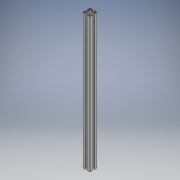
# Autodesk Inventor part: Alu_Proil_40
Saved by Autodesk Inventor 2019 (Build 230136000, 136)
## iProperties
Created: 2016-05-09
Part Number: Alu_Proil_40
Material: Generic
Document SubType Name: Modeling
Designer: Alfa
Density: 1 g/cm^3
Appearance: Default
Author: Alfa
Autodesk Inventor part; units mm, degrees
ref_plane "YZ Plane" through (0, 0, 0) normal (1, 0, 0) x (0, 1, 0)
ref_plane "XZ Plane" through (0, 0, 0) normal (0, 1, 0) x (-1, 0, 0)
ref_plane "XY Plane" through (0, 0, 0) normal (0, 0, 1) x (1, 0, 0)
sketch "Sketch1" plane through (0, 0, 0) normal (0, 0, 1) x (1, 0, 0)
  circle A0 centre (0, 0) radius 3.4
  line L0 (12.55, 11.55) -> (17.5, 11.55)
  arc A1 (17.5, 11.55) -> (18.5, 12.55) centre (17.5, 12.55) ccw
  line L1 (18.5, 12.55) -> (18.5, 15.5)
  arc A2 (18.5, 15.5) -> (17.6213, 17.6213) centre (15.5, 15.5) ccw
  arc A3 (17.6213, 17.6213) -> (15.5, 18.5) centre (15.5, 15.5) ccw
  line L2 (15.5, 18.5) -> (12.55, 18.5)
  arc A4 (12.55, 18.5) -> (11.55, 17.5) centre (12.55, 17.5) ccw
  line L3 (11.55, 17.5) -> (11.55, 12.55)
  arc A5 (11.55, 12.55) -> (11.8429, 11.8429) centre (12.55, 12.55) ccw
  arc A6 (11.8429, 11.8429) -> (12.55, 11.55) centre (12.55, 12.55) ccw
  line L4 (-11.55, 12.55) -> (-11.55, 17.5)
  arc A7 (-11.55, 17.5) -> (-12.55, 18.5) centre (-12.55, 17.5) ccw
  line L5 (-12.55, 18.5) -> (-15.5, 18.5)
  arc A8 (-15.5, 18.5) -> (-17.6213, 17.6213) centre (-15.5, 15.5) ccw
  arc A9 (-17.6213, 17.6213) -> (-18.5, 15.5) centre (-15.5, 15.5) ccw
  line L6 (-18.5, 15.5) -> (-18.5, 12.55)
  arc A10 (-18.5, 12.55) -> (-17.5, 11.55) centre (-17.5, 12.55) ccw
  line L7 (-17.5, 11.55) -> (-12.55, 11.55)
  arc A11 (-12.55, 11.55) -> (-11.8429, 11.8429) centre (-12.55, 12.55) ccw
  arc A12 (-11.8429, 11.8429) -> (-11.55, 12.55) centre (-12.55, 12.55) ccw
  line L8 (-12.55, -11.55) -> (-17.5, -11.55)
  arc A13 (-17.5, -11.55) -> (-18.5, -12.55) centre (-17.5, -12.55) ccw
  line L9 (-18.5, -12.55) -> (-18.5, -15.5)
  arc A14 (-18.5, -15.5) -> (-17.6213, -17.6213) centre (-15.5, -15.5) ccw
  arc A15 (-17.6213, -17.6213) -> (-15.5, -18.5) centre (-15.5, -15.5) ccw
  line L10 (-15.5, -18.5) -> (-12.55, -18.5)
  arc A16 (-12.55, -18.5) -> (-11.55, -17.5) centre (-12.55, -17.5) ccw
  line L11 (-11.55, -17.5) -> (-11.55, -12.55)
  arc A17 (-11.55, -12.55) -> (-11.8429, -11.8429) centre (-12.55, -12.55) ccw
  arc A18 (-11.8429, -11.8429) -> (-12.55, -11.55) centre (-12.55, -12.55) ccw
  line L12 (11.55, -12.55) -> (11.55, -17.5)
  arc A19 (11.55, -17.5) -> (12.55, -18.5) centre (12.55, -17.5) ccw
  line L13 (12.55, -18.5) -> (15.5, -18.5)
  arc A20 (15.5, -18.5) -> (17.6213, -17.6213) centre (15.5, -15.5) ccw
  arc A21 (17.6213, -17.6213) -> (18.5, -15.5) centre (15.5, -15.5) ccw
  line L14 (18.5, -15.5) -> (18.5, -12.55)
  arc A22 (18.5, -12.55) -> (17.5, -11.55) centre (17.5, -12.55) ccw
  line L15 (17.5, -11.55) -> (12.55, -11.55)
  arc A23 (12.55, -11.55) -> (11.8429, -11.8429) centre (12.55, -12.55) ccw
  arc A24 (11.8429, -11.8429) -> (11.55, -12.55) centre (12.55, -12.55) ccw
  line L16 (-5.1, -19.8) -> (-5.1, -19)
  line L17 (-5.1, -19) -> (-4.1, -19)
  line L18 (-4.1, -19) -> (-4.1, -15.5)
  line L19 (-4.1, -15.5) -> (-6.4, -15.5)
  line L20 (-6.4, -15.5) -> (-6.4, -17.2)
  arc A25 (-7.4, -18.2) -> (-6.4, -17.2) centre (-7.4, -17.2) ccw
  line L21 (-7.4, -18.2) -> (-9.25, -18.2)
  arc A26 (-10.25, -17.2) -> (-9.25, -18.2) centre (-9.25, -17.2) ccw
  line L22 (-10.25, -17.2) -> (-10.25, -12.4926)
  arc A27 (-9.6642, -11.0784) -> (-10.25, -12.4926) centre (-8.25, -12.4926) ccw
  line L23 (-9.6642, -11.0784) -> (-5.1716, -6.5858)
  arc A28 (-3.7574, -6) -> (-5.1716, -6.5858) centre (-3.7574, -8) ccw
  line L24 (-3.7574, -6) -> (0, -6)
  line L25 (0, -6) -> (3.7574, -6)
  arc A29 (5.1716, -6.5858) -> (3.7574, -6) centre (3.7574, -8) ccw
  line L26 (5.1716, -6.5858) -> (9.6642, -11.0784)
  arc A30 (10.25, -12.4926) -> (9.6642, -11.0784) centre (8.25, -12.4926) ccw
  line L27 (10.25, -12.4926) -> (10.25, -17.2)
  arc A31 (9.25, -18.2) -> (10.25, -17.2) centre (9.25, -17.2) ccw
  line L28 (9.25, -18.2) -> (7.4, -18.2)
  arc A32 (6.4, -17.2) -> (7.4, -18.2) centre (7.4, -17.2) ccw
  line L29 (6.4, -17.2) -> (6.4, -15.5)
  line L30 (6.4, -15.5) -> (4.1, -15.5)
  line L31 (4.1, -15.5) -> (4.1, -19)
  line L32 (4.1, -19) -> (5.1, -19)
  line L33 (5.1, -19) -> (5.1, -19.8)
  arc A33 (5.1, -19.8) -> (5.3, -20) centre (5.3, -19.8) ccw
  line L34 (5.3, -20) -> (15.5, -20)
  arc A34 (15.5, -20) -> (18.682, -18.682) centre (15.5, -15.5) ccw
  arc A35 (18.682, -18.682) -> (20, -15.5) centre (15.5, -15.5) ccw
  line L35 (20, -15.5) -> (20, -5.3)
  arc A36 (20, -5.3) -> (19.8, -5.1) centre (19.8, -5.3) ccw
  line L36 (19.8, -5.1) -> (19, -5.1)
  line L37 (19, -5.1) -> (19, -4.1)
  line L38 (19, -4.1) -> (15.5, -4.1)
  line L39 (15.5, -4.1) -> (15.5, -6.4)
  line L40 (15.5, -6.4) -> (17.2, -6.4)
  arc A37 (18.2, -7.4) -> (17.2, -6.4) centre (17.2, -7.4) ccw
  line L41 (18.2, -7.4) -> (18.2, -9.25)
  arc A38 (17.2, -10.25) -> (18.2, -9.25) centre (17.2, -9.25) ccw
  line L42 (17.2, -10.25) -> (12.4926, -10.25)
  arc A39 (11.0784, -9.6642) -> (12.4926, -10.25) centre (12.4926, -8.25) ccw
  line L43 (11.0784, -9.6642) -> (6.5858, -5.1716)
  arc A40 (6, -3.7574) -> (6.5858, -5.1716) centre (8, -3.7574) ccw
  line L44 (6, -3.7574) -> (6, 0)
  line L45 (6, 0) -> (6, 3.7574)
  arc A41 (6.5858, 5.1716) -> (6, 3.7574) centre (8, 3.7574) ccw
  line L46 (6.5858, 5.1716) -> (11.0784, 9.6642)
  arc A42 (12.4926, 10.25) -> (11.0784, 9.6642) centre (12.4926, 8.25) ccw
  line L47 (12.4926, 10.25) -> (17.2, 10.25)
  arc A43 (18.2, 9.25) -> (17.2, 10.25) centre (17.2, 9.25) ccw
  line L48 (18.2, 9.25) -> (18.2, 7.4)
  arc A44 (17.2, 6.4) -> (18.2, 7.4) centre (17.2, 7.4) ccw
  line L49 (17.2, 6.4) -> (15.5, 6.4)
  line L50 (15.5, 6.4) -> (15.5, 4.1)
  line L51 (15.5, 4.1) -> (19, 4.1)
  line L52 (19, 4.1) -> (19, 5.1)
  line L53 (19, 5.1) -> (19.8, 5.1)
  arc A45 (19.8, 5.1) -> (20, 5.3) centre (19.8, 5.3) ccw
  line L54 (20, 5.3) -> (20, 15.5)
  arc A46 (20, 15.5) -> (18.682, 18.682) centre (15.5, 15.5) ccw
  arc A47 (18.682, 18.682) -> (15.5, 20) centre (15.5, 15.5) ccw
  line L55 (15.5, 20) -> (5.3, 20)
  arc A48 (5.3, 20) -> (5.1, 19.8) centre (5.3, 19.8) ccw
  line L56 (5.1, 19.8) -> (5.1, 19)
  line L57 (5.1, 19) -> (4.1, 19)
  line L58 (4.1, 19) -> (4.1, 15.5)
  line L59 (4.1, 15.5) -> (6.4, 15.5)
  line L60 (6.4, 15.5) -> (6.4, 17.2)
  arc A49 (7.4, 18.2) -> (6.4, 17.2) centre (7.4, 17.2) ccw
  line L61 (7.4, 18.2) -> (9.25, 18.2)
  arc A50 (10.25, 17.2) -> (9.25, 18.2) centre (9.25, 17.2) ccw
  line L62 (10.25, 17.2) -> (10.25, 12.4926)
  arc A51 (9.6642, 11.0784) -> (10.25, 12.4926) centre (8.25, 12.4926) ccw
  line L63 (9.6642, 11.0784) -> (5.1716, 6.5858)
  arc A52 (3.7574, 6) -> (5.1716, 6.5858) centre (3.7574, 8) ccw
  line L64 (3.7574, 6) -> (0, 6)
  line L65 (0, 6) -> (-3.7574, 6)
  arc A53 (-5.1716, 6.5858) -> (-3.7574, 6) centre (-3.7574, 8) ccw
  line L66 (-5.1716, 6.5858) -> (-9.6642, 11.0784)
  arc A54 (-10.25, 12.4926) -> (-9.6642, 11.0784) centre (-8.25, 12.4926) ccw
  line L67 (-10.25, 12.4926) -> (-10.25, 17.2)
  arc A55 (-9.25, 18.2) -> (-10.25, 17.2) centre (-9.25, 17.2) ccw
  line L68 (-9.25, 18.2) -> (-7.4, 18.2)
  arc A56 (-6.4, 17.2) -> (-7.4, 18.2) centre (-7.4, 17.2) ccw
  line L69 (-6.4, 17.2) -> (-6.4, 15.5)
  line L70 (-6.4, 15.5) -> (-4.1, 15.5)
  line L71 (-4.1, 15.5) -> (-4.1, 19)
  line L72 (-4.1, 19) -> (-5.1, 19)
  line L73 (-5.1, 19) -> (-5.1, 19.8)
  arc A57 (-5.1, 19.8) -> (-5.3, 20) centre (-5.3, 19.8) ccw
  line L74 (-5.3, 20) -> (-15.5, 20)
  arc A58 (-15.5, 20) -> (-18.682, 18.682) centre (-15.5, 15.5) ccw
  arc A59 (-18.682, 18.682) -> (-20, 15.5) centre (-15.5, 15.5) ccw
  line L75 (-20, 15.5) -> (-20, 5.3)
  arc A60 (-20, 5.3) -> (-19.8, 5.1) centre (-19.8, 5.3) ccw
  line L76 (-19.8, 5.1) -> (-19, 5.1)
  line L77 (-19, 5.1) -> (-19, 4.1)
  line L78 (-19, 4.1) -> (-15.5, 4.1)
  line L79 (-15.5, 4.1) -> (-15.5, 6.4)
  line L80 (-15.5, 6.4) -> (-17.2, 6.4)
  arc A61 (-18.2, 7.4) -> (-17.2, 6.4) centre (-17.2, 7.4) ccw
  line L81 (-18.2, 7.4) -> (-18.2, 9.25)
  arc A62 (-17.2, 10.25) -> (-18.2, 9.25) centre (-17.2, 9.25) ccw
  line L82 (-17.2, 10.25) -> (-12.4926, 10.25)
  arc A63 (-11.0784, 9.6642) -> (-12.4926, 10.25) centre (-12.4926, 8.25) ccw
  line L83 (-11.0784, 9.6642) -> (-6.5858, 5.1716)
  arc A64 (-6, 3.7574) -> (-6.5858, 5.1716) centre (-8, 3.7574) ccw
  line L84 (-6, 3.7574) -> (-6, 0)
  line L85 (-6, 0) -> (-6, -3.7574)
  arc A65 (-6.5858, -5.1716) -> (-6, -3.7574) centre (-8, -3.7574) ccw
  line L86 (-6.5858, -5.1716) -> (-11.0784, -9.6642)
  arc A66 (-12.4926, -10.25) -> (-11.0784, -9.6642) centre (-12.4926, -8.25) ccw
  line L87 (-12.4926, -10.25) -> (-17.2, -10.25)
  arc A67 (-18.2, -9.25) -> (-17.2, -10.25) centre (-17.2, -9.25) ccw
  line L88 (-18.2, -9.25) -> (-18.2, -7.4)
  arc A68 (-17.2, -6.4) -> (-18.2, -7.4) centre (-17.2, -7.4) ccw
  line L89 (-17.2, -6.4) -> (-15.5, -6.4)
  line L90 (-15.5, -6.4) -> (-15.5, -4.1)
  line L91 (-15.5, -4.1) -> (-19, -4.1)
  line L92 (-19, -4.1) -> (-19, -5.1)
  line L93 (-19, -5.1) -> (-19.8, -5.1)
  arc A69 (-19.8, -5.1) -> (-20, -5.3) centre (-19.8, -5.3) ccw
  line L94 (-20, -5.3) -> (-20, -15.5)
  arc A70 (-20, -15.5) -> (-18.682, -18.682) centre (-15.5, -15.5) ccw
  arc A71 (-18.682, -18.682) -> (-15.5, -20) centre (-15.5, -15.5) ccw
  line L95 (-15.5, -20) -> (-5.3, -20)
  arc A72 (-5.3, -20) -> (-5.1, -19.8) centre (-5.3, -19.8) ccw
  dimension "d0" = 4.1
  dimension "d1" = 5.1
  dimension "d2" = 6.4
  dimension "d3" = 7.4
  dimension "d4" = 9.25
  dimension "d5" = 10.25
  dimension "d6" = 11.55
  dimension "d7" = 12.55
  dimension "d8" = 15.5
  dimension "d9" = 18.5
  dimension "d10" = 20
  dimension "d11" = 17.5
  dimension "d15" = 6.8
  constraints: 192 end point, 178 tangent, 144 point on circle, 73 centre point, 54 equal radius, 46 parallel, 23 perpendicular, 2 collinear
  measures "d0" distance from line of A0.centre L58
  measures "d1" distance from line of A0.centre L56
  measures "d2" horizontal distance of A0.centre L59.end
  measures "d3" horizontal distance of A0.centre A49.centre
  measures "d4" horizontal distance of A0.centre A50.centre
  measures "d5" distance from line of A0.centre L62
  measures "d6" distance from line of A0.centre L3
  measures "d7" horizontal distance of A0.centre A4.centre
  measures "d8" horizontal distance of A0.centre A2.centre
  measures "d9" distance from line of A0.centre L1
  measures "d10" distance from line of A0.centre L54
  measures "d11" horizontal distance of A0.centre A1.centre
  measures "d15" diameter of A0
extrude "Extrusion1" add sketch "Sketch1" along normal blind 700
body "Solid1"
